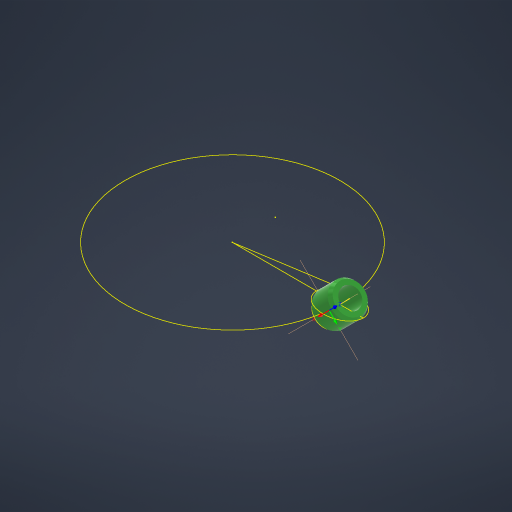
# Autodesk Inventor part: Roller
Saved by Autodesk Inventor 2023.1 (Build 271208000, 208)
## iProperties
Created: 2022-11-26
Part Number: Roller
Material: PC/ABS Plastic
Document SubType Name: Modeling
Designer: aubrey-work
Density: 0.357273 g/cm^3
Appearance: Smooth - Dark Forest Green
Author: aubrey-work
Autodesk Inventor part; units mm, degrees
ref_plane "YZ Plane" through (0, 0, 0) normal (1, 0, 0) x (0, 1, 0)
ref_plane "XZ Plane" through (0, 0, 0) normal (0, 1, 0) x (-1, 0, 0)
ref_plane "XY Plane" through (0, 0, 0) normal (0, 0, 1) x (1, 0, 0)
derived "Slew Bearing Master.ipt"
sketch "Sketch1" plane through (0, 0, 0) normal (0, 1, 0) x (-1, 0, 0)
  circle A0 centre (0, 0) radius 26.2043
  ellipse E0 centre (-26.2043, 0) end of major axis (-31.9319, 0) minor radius 4.05
  line L0 (-20.4767, 0) -> (-31.9319, 0)
  line L1 (-26.2043, -4.05) -> (-26.2043, 4.05)
  line L2 (0, 0) -> (-26.2043, 0)
  line L3 (0, 0) -> (-24.9524, -3.9521)
sketch "Sketch2" plane through (0, 0, 0) normal (0, 0, 1) x (1, 0, 0)
  line L0 (31.9319, 0) -> (20.4767, 0)
  line L1 (20.4767, 0) -> (26.2043, -5.7276)
  line L2 (26.2043, -5.7276) -> (31.9319, 0)
  line L3 (31.9319, 0) -> (26.2043, 5.7276)
  line L4 (26.2043, 5.7276) -> (20.4767, 0)
  line L5 (23.3405, 2.8638) -> (29.0681, -2.8638)
  line L6 (23.3405, -2.8638) -> (29.0681, 2.8638)
  line L7 (26.2043, 5.7276) -> (26.2043, -5.7276)
  line L8 (27.0642, -4.797) -> (31.0013, -0.8599)
  line L9 (31.0013, -0.8599) -> (31.2601, 0.1061)
  line L10 (31.2601, 0.1061) -> (30.4823, 0.8839)
  line L11 (30.4823, 0.8839) -> (25.3204, -4.278)
  line L12 (25.3204, -4.278) -> (26.0982, -5.0558)
  line L13 (26.0982, -5.0558) -> (27.0642, -4.797)
  point P0 (0, 0)
revolve "Revolution2" add sketch "Sketch2" angle 360 about axis through (23.3405, -2.8638, 0) along (0.7071068, 0.7071068, 0) contours L9 L8 L5 L11 L0 | L0 L11 L10 L9 | L8 L13 L7 L11 L5 | L13 L12 L11 L7
sketch "UCS" plane through (23.6234, -2.5809, 0) normal (-0.7071068, -0.7071068, 0) x (-0.7071068, 0.7071068, 0)
  circle A0 centre (0, 0) radius 3.5 projected
  line L0 (3.5, 0) -> (-3.5, 0) construction
  line L1 (0, 3.5) -> (0, -3.5) construction
  point P0 (18.5292, 0)
  constraints: 4 end point, 4 point on circle, 1 horizontal, 1 perpendicular
equation "\"gap\" = 0.1"
equation "\"airgap\" = 0.4"
equation "\"wallgap\" = 2"
equation "\"roller_outerDiameter\" = 8"
equation "\"roller_diameter\" = 8"
